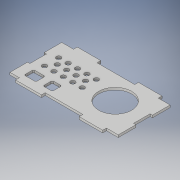
# Autodesk Inventor part: Part Sisi 2
Saved by Autodesk Inventor 2019 (Build 230136000, 136)
## iProperties
Created: 2019-07-08
Part Number: Part Sisi 2
Material: Generic
Document SubType Name: Modeling
Designer: azriel
Density: 1 g/cm^3
Appearance: Default
Author: azriel
Autodesk Inventor part; units mm, degrees
ref_plane "YZ Plane" through (0, 0, 0) normal (1, 0, 0) x (0, 1, 0)
ref_plane "XZ Plane" through (0, 0, 0) normal (0, 1, 0) x (-1, 0, 0)
ref_plane "XY Plane" through (0, 0, 0) normal (0, 0, 1) x (1, 0, 0)
sketch "Sketch1" plane through (0, 0, 0) normal (0, 1, 0) x (-1, 0, 0)
  line L0 (42.6597, 73.3147) -> (42.6597, 81.3147)
  line L1 (42.6597, 81.3147) -> (97.6597, 81.3147)
  line L2 (97.6597, 81.3147) -> (97.6597, 73.3147)
  line L3 (-87.3403, 73.3147) -> (-87.3403, 81.3147)
  line L4 (-87.3403, 81.3147) -> (-37.3403, 81.3147)
  line L5 (-37.3403, 81.3147) -> (-37.3403, 73.3147)
  line L6 (117.6597, 73.3147) -> (97.6597, 73.3147)
  line L7 (42.6597, 73.3147) -> (-37.3403, 73.3147)
  line L8 (-87.3403, 73.3147) -> (-112.3403, 73.3147)
  line L9 (127.6597, 35.8147) -> (132.6597, 35.8147)
  line L10 (132.6597, 73.3147) -> (127.6597, 73.3147)
  line L11 (97.6597, 46.3147) -> (97.6597, 60.3147)
  line L12 (94.6597, 63.3147) -> (75.6597, 63.3147)
  line L13 (72.6597, 60.3147) -> (72.6597, 46.3147)
  line L14 (75.6597, 43.3147) -> (94.6597, 43.3147)
  line L15 (54.6597, 63.3147) -> (40.6597, 63.3147)
  line L16 (37.6597, 60.3147) -> (37.6597, 46.3147)
  line L17 (40.6597, 43.3147) -> (54.6597, 43.3147)
  line L18 (57.6597, 46.3147) -> (57.6597, 60.3147)
  circle A0 centre (52.6374, -5.1409) radius 5
  circle A1 centre (32.6374, -5.1409) radius 5
  circle A2 centre (12.6374, -5.1409) radius 5
  circle A3 centre (72.6374, -5.1409) radius 5
  circle A4 centre (92.6374, -5.1409) radius 5
  circle A5 centre (21.6374, 8.8594) radius 5
  circle A6 centre (41.6374, 8.8594) radius 5
  circle A7 centre (61.6374, 8.8594) radius 5
  circle A8 centre (81.6374, 8.8594) radius 5
  circle A9 centre (52.6374, 24.8594) radius 5
  circle A10 centre (32.6374, 24.8594) radius 5
  circle A11 centre (12.6374, 24.8594) radius 5
  circle A12 centre (72.6374, 24.8594) radius 5
  circle A13 centre (92.6374, 24.8594) radius 5
  circle A14 centre (-46.3382, 13.8594) radius 35
  arc A15 (72.6597, 46.3147) -> (75.6597, 43.3147) centre (75.6597, 46.3147) ccw
  arc A16 (94.6597, 43.3147) -> (97.6597, 46.3147) centre (94.6597, 46.3147) ccw
  arc A17 (97.6597, 60.3147) -> (94.6597, 63.3147) centre (94.6597, 60.3147) ccw
  arc A18 (75.6597, 63.3147) -> (72.6597, 60.3147) centre (75.6597, 60.3147) ccw
  arc A19 (54.6597, 43.3147) -> (57.6597, 46.3147) centre (54.6597, 46.3147) ccw
  arc A20 (57.6597, 60.3147) -> (54.6597, 63.3147) centre (54.6597, 60.3147) ccw
  arc A21 (40.6597, 63.3147) -> (37.6597, 60.3147) centre (40.6597, 60.3147) ccw
  arc A22 (37.6597, 46.3147) -> (40.6597, 43.3147) centre (40.6597, 46.3147) ccw
  line L19 (42.6374, -36.6853) -> (42.6374, -44.6853)
  line L20 (42.6374, -44.6853) -> (92.6374, -44.6853)
  line L21 (92.6374, -44.6853) -> (92.6374, -36.6853)
  line L22 (-87.3403, -36.6853) -> (-87.3403, -44.6853)
  line L23 (-87.3403, -44.6853) -> (-37.3403, -44.6853)
  line L24 (-37.3403, -44.6853) -> (-37.3403, -36.6853)
  line L25 (-112.3403, -36.6853) -> (-87.3403, -36.6853)
  line L26 (-37.3403, -36.6853) -> (42.6374, -36.6853)
  line L27 (92.6374, -36.6853) -> (112.6597, -36.6853)
  line L28 (112.6597, 0.8147) -> (117.6597, 0.8147)
  line L29 (117.6597, 0.8147) -> (117.6597, -36.6853)
  line L30 (117.6597, -36.6853) -> (112.6597, -36.6853)
  line L31 (112.6597, 35.8147) -> (117.6597, 35.8147)
  line L32 (117.6597, 35.8147) -> (117.6597, 73.3147)
  line L33 (117.6597, 73.3147) -> (117.6597, 73.3147)
  line L34 (112.6597, 0.8147) -> (112.6597, 35.8147)
  line L35 (-112.3403, 0.8147) -> (-112.3403, -36.6853)
  line L36 (-112.3403, 0.8147) -> (-107.3403, 0.8147)
  line L37 (-107.3403, 0.8147) -> (-107.3403, 35.8147)
  line L38 (-107.3403, 35.8147) -> (-112.3403, 35.8147)
  line L39 (-112.3403, 35.8147) -> (-112.3403, 73.3147)
  point P0 (0, 0)
  point P1 (97.6597, 43.3147)
  point P2 (97.6597, 63.3147)
  point P3 (72.6597, 63.3147)
  point P4 (72.6597, 43.3147)
  point P5 (57.6597, 63.3147)
  point P6 (37.6597, 63.3147)
  point P7 (37.6597, 43.3147)
  point P8 (57.6597, 43.3147)
  point P9 (97.6597, 45.3147)
  point P10 (95.6597, 43.3147)
  point P11 (110.6597, 63.3147)
  point P12 (97.6597, 61.3147)
  point P13 (89.6597, 63.3147)
  point P14 (72.6597, 61.3147)
  point P15 (72.6597, 45.3147)
  point P16 (74.6597, 43.3147)
  point P17 (57.6597, 45.3147)
  point P18 (55.6597, 43.3147)
  point P19 (39.6597, 43.3147)
  point P20 (37.6597, 45.3147)
  point P21 (39.6597, 63.3147)
  point P22 (37.6597, 61.3147)
  point P23 (55.6597, 63.3147)
  point P24 (57.6597, 61.3147)
  dimension "d1" = 240
  dimension "d3" = 8
  dimension "d5" = 8
  dimension "d6" = 80
  dimension "d20" = 20
  dimension "d21" = 25
  dimension "d22" = 10
  dimension "d29" = 20
  dimension "d31" = 15
  dimension "d64" = 70
  dimension "d68" = 3
  dimension "d69" = 3
  dimension "d70" = 3
  dimension "d71" = 3
  dimension "d73" = 50
  dimension "d74" = 8
  dimension "d75" = 50
  dimension "d76" = 8
  dimension "d81" = 5
  dimension "d82" = 5
  dimension "d86" = 20
  dimension "d89" = 5
  constraints: 80 end point, 32 point on line, 23 centre point, 16 point on circle, 16 tangent, 15 parallel, 10 perpendicular, 5 horizontal, 4 equal radius, 1 vertical
  measures "d1" distance of L8.end L10.end
  measures "d3" distance of L0.start L0.end
  measures "d5" distance of L3.start L3.end
  measures "d6" distance between parallel lines of L0 L5
  measures "d20" distance of point (97.66, 43.315) point (97.66, 63.315)
  measures "d21" distance of point (72.66, 63.315) point (97.66, 63.315)
  measures "d22" distance between parallel lines of L6 L12
  measures "d29" distance of point (57.66, 63.315) point (37.66, 63.315)
  measures "d31" distance between parallel lines of L18 L13
  measures "d64" diameter of A14
  measures "d68" radius of A15
  measures "d69" radius of A16
  measures "d70" radius of A17
  measures "d71" radius of A19
  measures "d73" distance of L21.end L19.start
  measures "d74" distance of L19.end L19.start
  measures "d75" distance of L24.end L22.start
  measures "d76" distance of L22.end L22.start
  measures "d81" distance of L28.start L28.end
  measures "d82" distance of L31.start L31.end
  measures "d86" distance between parallel lines of L11 L32
  measures "d89" distance of L35.start L36.end
extrude "Extrusion2" add sketch "Sketch1" along normal blind 5
body "Solid2"
